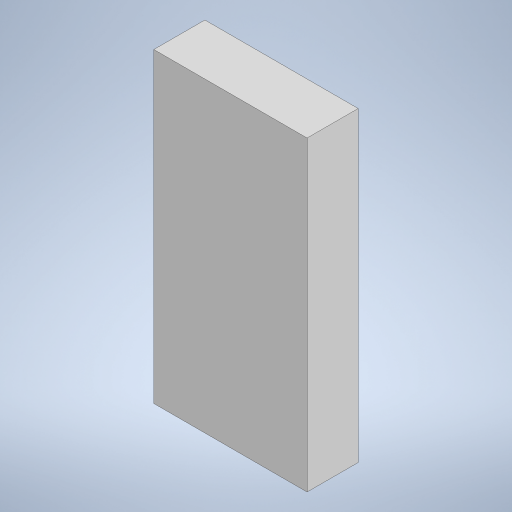
# Autodesk Inventor part: Motor Brace
Saved by Autodesk Inventor 2024 (Build 280153000, 153)
## iProperties
Created: 2025-01-21
Part Number: Motor Brace
Material: Generic
Document SubType Name: Modeling
Designer: Sven
Density: 1 g/cm^3
Appearance: Default
Author: Sven
Autodesk Inventor part; units mm, degrees
ref_plane "YZ Plane" through (0, 0, 0) normal (1, 0, 0) x (0, 1, 0)
ref_plane "XZ Plane" through (0, 0, 0) normal (0, 1, 0) x (-1, 0, 0)
ref_plane "XY Plane" through (0, 0, 0) normal (0, 0, 1) x (1, 0, 0)
sketch "Sketch1" plane through (0, 0, 0) normal (0, 0, 1) x (1, 0, 0)
  line L0 (-19.05, 38.1) -> (19.05, 38.1)
  line L1 (19.05, 38.1) -> (19.05, -38.1)
  line L2 (19.05, -38.1) -> (-19.05, -38.1)
  line L3 (-19.05, -38.1) -> (-19.05, 38.1)
  point P0 (0, 0)
  point P1 (19.05, 0)
  point P2 (0, 38.1)
  dimension "d0" = 38.1
  dimension "d1" = 76.2
  constraints: 8 end point, 2 midpoint, 2 parallel, 1 horizontal, 1 horizontal alignment, 1 perpendicular, 1 vertical alignment
  measures "d0" distance of L0.start L0.end
  measures "d1" distance of L0.end L1.end
extrude "Extrusion1" add sketch "Sketch1" along normal blind 12.7
body "Solid1"
